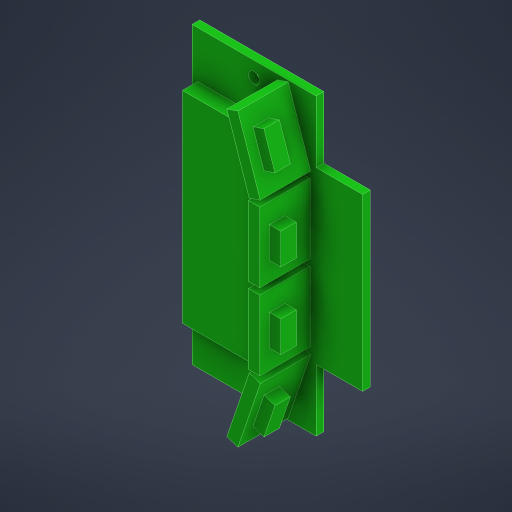
# Autodesk Inventor part: płytka_pcb
Saved by Autodesk Inventor 2023.4 (Build 274418000, 418)
## iProperties
Created: 2025-10-31
Part Number: płytka_pcb
Material: Tworzywo sztuczne ABS
Document SubType Name: Modeling
Designer: Jakub Borsukiewicz
Density: 1.06 g/cm^3
Appearance: Ciemnozielona
Author: Jakub Borsukiewicz
Autodesk Inventor part; units mm, degrees
ref_plane "YZ Plane" through (0, 0, 0) normal (1, 0, 0) x (0, 1, 0)
ref_plane "XZ Plane" through (0, 0, 0) normal (0, 1, 0) x (-1, 0, 0)
ref_plane "XY Plane" through (0, 0, 0) normal (0, 0, 1) x (1, 0, 0)
sketch "Szkic1" plane through (0, 0, 0) normal (0, 0, 1) x (1, 0, 0)
  line L0 (0, -7.6) -> (0, 45.6) projected
  line L1 (-8.8, 0) -> (52.8, 0) projected
  line L2 (0, 0) -> (32, 0)
  line L3 (32, 0) -> (32, 38)
  line L4 (32, 38) -> (0, 38)
  line L5 (0, 38) -> (0, 0)
  circle A0 centre (16, 34) radius 1.5
  line L6 (32, 0) -> (44, 0)
  line L7 (44, 0) -> (44, 22)
  line L8 (44, 22) -> (32, 22)
  line L9 (32, 22) -> (32, 0)
  point P0 (0, 38)
  point P1 (32, 0)
  dimension "d0" = 32
  dimension "d1" = 38
  dimension "d2" = 3
  dimension "d3" = 4
  dimension "d4" = 16
  dimension "d18" = 12
  dimension "d19" = 22
  constraints: 16 end point, 4 parallel, 2 horizontal, 2 perpendicular, 1 centre point
  measures "d0" distance of L3.end L4.end
  measures "d1" distance of L2.end L3.end
  measures "d2" diameter of A0
  measures "d3" distance from line of L4 A0.centre
  measures "d4" distance from line of L5 A0.centre
  measures "d18" distance of L8.end L7.end
  measures "d19" distance of L6.end L7.end
extrude "Wyciągnięcie proste1" add sketch "Szkic1" along normal blind 2
sketch "Szkic2" plane through (0, 0, 2) normal (0, 0, 1) x (1, 0, 0)
  line L0 (0, 38) -> (0, 0) projected
  line L1 (0, 0) -> (44, 0) projected
  line L2 (32, 22) -> (32, 38) projected
  line L3 (32, 38) -> (0, 38) projected
  circle A0 centre (16, 34) radius 1.5 projected
  line L4 (0, 0) -> (44, 0) projected
  line L5 (1.5, 0) -> (22.5, 0)
  line L6 (22.5, 0) -> (22.5, 26)
  line L7 (22.5, 26) -> (1.5, 26)
  line L8 (1.5, 26) -> (1.5, 0)
  line L9 (44, 0) -> (44, 22) projected
  line L10 (44, 22) -> (32, 22) projected
  point P0 (32, 0)
  dimension "d7" = 26
  dimension "d8" = 21
  dimension "d9" = 1.5
  constraints: 8 end point, 2 parallel, 1 horizontal, 1 perpendicular, 1 point on line
  measures "d7" distance of L5.end L6.end
  measures "d8" distance of L6.end L7.end
  measures "d9" distance between parallel lines of L0 L8
extrude "Wyciągnięcie proste2" add sketch "Szkic2" along normal blind 4 contours L8 L7 L6 L1
sketch "Szkic3" plane through (0, 0, 2) normal (0, 0, 1) x (1, 0, 0)
  line L0 (27.4645, 18.8335) -> (30.4645, 18.8335)
  line L1 (30.4645, 18.8335) -> (30.4645, 0.8335)
  line L2 (30.4645, 0.8335) -> (27.4645, 0.8335)
  line L3 (27.4645, 0.8335) -> (27.4645, 18.8335)
  line L4 (32, 22) -> (32, 38) projected
  line L5 (21.9813, 36.596) -> (24.8234, 37.5566)
  line L6 (24.8234, 37.5566) -> (30.5867, 20.5042)
  line L7 (30.5867, 20.5042) -> (27.7447, 19.5436)
  line L8 (27.7447, 19.5436) -> (21.9813, 36.596)
  point P0 (0, 0)
  point P1 (32, 0)
  point P2 (26, 22.676)
  point P3 (26, 4.676)
  dimension "d14" = 18
  dimension "d15" = 3
  dimension "d20" = 18
  dimension "d21" = 3
  constraints: 16 end point, 4 parallel, 3 perpendicular
  measures "d14" distance of L0.end L1.end
  measures "d15" distance of L1.end L2.end
  measures "d20" distance of L5.end L6.end
  measures "d21" distance of L5.start L5.end
extrude "Wyciągnięcie proste3" add sketch "Szkic3" along normal blind 13
sketch "Szkic4" plane through (30.4645, 0.8335, 2) normal (1, 0, 0) x (0, 0, -1)
  line L0 (0, 18) -> (0, 0) projected
  line L1 (0, 18) -> (-13, 18) projected
  line L2 (-13, 0) -> (-13, 18) projected
  line L3 (0, 0) -> (-13, 0) projected
  line L4 (-10.5669, 4.9788) -> (-6.5, 4.9788)
  line L5 (-6.5, 4.9788) -> (-6.5, 12.9492)
  line L6 (-6.5, 12.9492) -> (-10.5669, 12.9492)
  line L7 (-10.5669, 12.9492) -> (-10.5669, 4.9788)
  point P0 (2, -0.8335)
  constraints: 8 end point, 2 parallel, 1 horizontal, 1 perpendicular
extrude "Wyciągnięcie proste4" add sketch "Szkic4" along normal blind 3 contours L7 L6 L5 L4
sketch "Szkic5" plane through (24.8234, 37.5566, 15) normal (0.9473547, 0.320186, 0) x (0, 0, -1)
  line L0 (13, 0) -> (13, -18) projected
  line L1 (13, 0) -> (0, 0) projected
  line L2 (0, -18) -> (0, 0) projected
  line L3 (13, -18) -> (0, -18) projected
  line L4 (2.5137, -13.1873) -> (6.5, -13.1873)
  line L5 (6.5, -13.1873) -> (6.5, -4.3066)
  line L6 (6.5, -4.3066) -> (2.5137, -4.3066)
  line L7 (2.5137, -4.3066) -> (2.5137, -13.1873)
  point P0 (15, -27.6313)
  constraints: 8 end point, 2 parallel, 1 horizontal, 1 perpendicular
extrude "Wyciągnięcie proste5" add sketch "Szkic5" along normal blind 3 contours L7 L6 L5 L4
mirror "Odbij2" about plane through (0, 0, 0) normal (0, 1, 0) of "Wyciągnięcie proste1", "Wyciągnięcie proste2", "Wyciągnięcie proste3", "Wyciągnięcie proste4", "Wyciągnięcie proste5"
